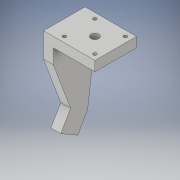
# Autodesk Inventor part: Stepper_Face
Saved by Autodesk Inventor 2019 (Build 230136000, 136)
## iProperties
Created: 2019-07-06
Part Number: Stepper_Face
Material: Generic
Document SubType Name: Modeling
Designer: Jorian Brusind
Density: 1 g/cm^3
Appearance: Default
Author: Jorian Brusind
Autodesk Inventor part; units mm, degrees
ref_plane "YZ Plane" through (0, 0, 0) normal (1, 0, 0) x (0, 1, 0)
ref_plane "XZ Plane" through (0, 0, 0) normal (0, 1, 0) x (-1, 0, 0)
ref_plane "XY Plane" through (0, 0, 0) normal (0, 0, 1) x (1, 0, 0)
sketch "Sketch1" plane through (0, 0, 0) normal (0, 1, 0) x (-1, 0, 0)
  line L0 (0, 0) -> (52.3, 0)
  line L1 (52.3, 0) -> (52.3, -42.3)
  line L2 (52.3, -42.3) -> (0, -42.3)
  line L3 (0, -42.3) -> (0, 0)
  dimension "d0" = 52.3
  dimension "d1" = 42.3
  constraints: 8 end point, 2 parallel, 1 horizontal, 1 perpendicular
  measures "d0" distance of L1.end L2.end
  measures "d1" distance of L0.end L1.end
extrude "Extrusion1" add sketch "Sketch1" along normal blind 10
sketch "Sketch2" plane through (0, 0, 0) normal (0, -1, 0) x (1, 0, 0)
  line L0 (-52.3, 0) -> (0, 0) projected
  line L1 (-52.3, 0) -> (-42.3, 0)
  line L2 (-42.3, 0) -> (-42.3, -42.3)
  line L3 (-42.3, -42.3) -> (-52.3, -42.3)
  line L4 (-52.3, -42.3) -> (-52.3, 0)
  dimension "d4" = 10
  dimension "d5" = 42.3
  constraints: 8 end point, 2 parallel, 1 horizontal, 1 perpendicular
  measures "d4" distance of L2.end L3.end
  measures "d5" distance of L1.end L2.end
extrude "Extrusion2" add sketch "Sketch2" along normal blind 15
sketch "Sketch3" plane through (0, 10, 0) normal (0, 1, 0) x (1, 0, 0)
  line L0 (0, 0) -> (0, 5.65)
  line L1 (0, 0) -> (0, 42.3) projected
  line L2 (0, 5.65) -> (-5.65, 5.65)
  circle A0 centre (-5.65, 5.65) radius 1.75
  circle A1 centre (-5.65, 36.65) radius 1.75
  circle A2 centre (-36.65, 5.65) radius 1.75
  circle A3 centre (-36.65, 36.65) radius 1.75
  dimension "d8" = 5.65
  dimension "d9" = 5.65
  dimension "d10" = 3.5
  dimension "d13" = 31
  dimension "d16" = 31
  constraints: 4 centre point, 4 end point, 1 coincident, 1 horizontal, 1 perpendicular, 1 point on line, 1 vertical, 6 other
  measures "d8" distance of L0.start L0.end
  measures "d9" distance of L0.end L2.end
  measures "d10" diameter of A0
  measures "d13" distance of A0.centre A1.centre
  measures "d16" distance of A0.centre A2.centre
extrude "Extrusion3" cut sketch "Sketch3" against normal blind 10
sketch "Sketch4" plane through (0, 10, 0) normal (0, 1, 0) x (1, 0, 0)
  line L0 (0, 42.3) -> (0, 0) projected
  line L1 (0, 21.15) -> (-21.15, 21.15)
  circle A0 centre (-21.15, 21.15) radius 4
  dimension "d21" = 21.15
  dimension "d22" = 8
  constraints: 2 end point, 1 centre point, 1 coincident, 1 horizontal, 1 midpoint
  measures "d21" distance of L1.start L1.end
  measures "d22" diameter of A0
extrude "Extrusion4" cut sketch "Sketch4" against normal blind 10
sketch "Sketch9" plane through (-52.3, 10, -42.3) normal (-1, 0, 0) x (0, 0, 1)
  line L0 (42.3, 0) -> (0, 0) projected
  line L1 (21.15, 0) -> (121.15, 0) construction
  line L2 (42.3, 0) -> (42.3, -25) projected
  line L3 (0, -25) -> (42.3, -25) projected
  line L4 (21.15, 0) -> (21.15, 14.2)
  line L5 (21.15, 14.2) -> (21.15, -85.8)
  line L6 (21.15, 14.2) -> (121.15, 14.2) construction
  line L7 (21.15, -85.8) -> (11.15, -85.8)
  line L8 (7.4897, -82.1397) -> (24.8103, -72.1397)
  line L9 (24.8103, -72.1397) -> (34.8103, -89.4603)
  line L10 (34.8103, -89.4603) -> (17.4897, -99.4603)
  line L11 (17.4897, -99.4603) -> (7.4897, -82.1397)
  line L12 (7.4897, -82.1397) -> (34.8103, -89.4603) construction
  line L13 (24.8103, -72.1397) -> (17.4897, -99.4603) construction
  line L14 (7.4897, -82.1397) -> (27.4897, -82.1397) construction
  line L15 (7.4897, -82.1397) -> (0, -25)
  line L16 (24.8103, -72.1397) -> (42.3, -25)
  point P0 (42.3, -10)
  dimension "d77" = 14.2
  dimension "d78" = 100
  dimension "d79" = 90
  dimension "d80" = 10
  dimension "d81" = 90
  dimension "d82" = 20
  dimension "d83" = 30
  dimension "d84" = 20
  constraints: 28 end point, 3 horizontal, 3 midpoint, 2 equal length, 2 parallel, 1 perpendicular, 1 vertical
  measures "d77" distance of L1.start L4.end
  measures "d78" distance of L4.end L5.end
  measures "d79" angle of L5 L6
  measures "d80" distance of L5.end L7.end
  measures "d81" angle of L5 L7
  measures "d82" distance of L8.start L8.end
  measures "d83" angle of L14 L8
  measures "d84" distance of L8.end L9.end
extrude "Extrusion8" add sketch "Sketch9" against normal blind 10 contours L16 L8 L5 L3 | L5 L8 L15 L3 | L9 L10 L11 L8
body "Solid1"
